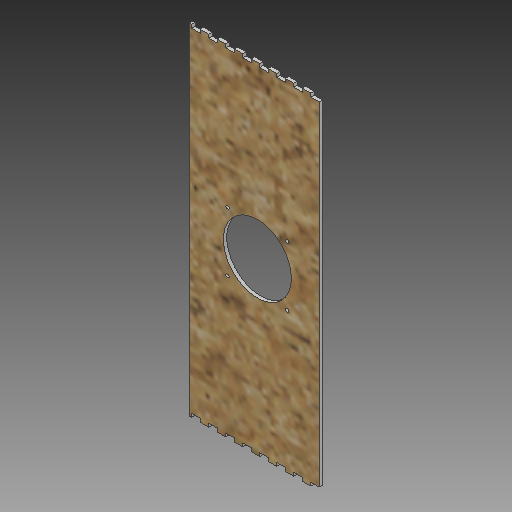
# Autodesk Inventor part: задняя стенка
Saved by Autodesk Inventor 2019 (Build 230136000, 136)
## iProperties
Created: 2022-06-28
Part Number: задняя стенка
Material: Типовые
Document SubType Name: Modeling
Designer: korsh
Density: 1 g/cm^3
Appearance: По умолчанию
Author: korsh
Autodesk Inventor part; units mm, degrees
ref_plane "YZ Plane" through (0, 0, 0) normal (1, 0, 0) x (0, 1, 0)
ref_plane "XZ Plane" through (0, 0, 0) normal (0, 1, 0) x (-1, 0, 0)
ref_plane "XY Plane" through (0, 0, 0) normal (0, 0, 1) x (1, 0, 0)
sketch "Эскиз1" plane through (0, 0, 0) normal (0, 0, 1) x (1, 0, 0)
  circle A0 centre (0, 0) radius 40 projected
  circle A1 centre (35, 35) radius 2 projected
  circle A2 centre (-35, 35) radius 2 projected
  circle A3 centre (-35, -35) radius 2 projected
  circle A4 centre (35, -35) radius 2 projected
  line L0 (72.777, 200) -> (-80, 200)
  line L1 (-80, 200) -> (-80, -200)
  line L2 (-80, -200) -> (72.777, -200)
  line L3 (72.777, -200) -> (72.777, 200)
  point P0 (0, 0)
  dimension "d0" = 400
  dimension "d1" = 200
  dimension "d2" = 80
  constraints: 8 end point, 2 parallel, 1 horizontal, 1 perpendicular
  measures "d0" distance of L2.end L0.start
  measures "d1" distance from line of point (0, 0) L2
  measures "d2" distance from line of L1 point (0, 0)
extrude "Выдавливание1" add sketch "Эскиз1" along normal blind 4
sketch "Эскиз3" plane through (0, 0, 4) normal (0, 0, 1) x (1, 0, 0)
  line L0 (72.777, 200) -> (62.777, 200)
  line L1 (62.777, 200) -> (62.777, 196)
  line L2 (62.777, 196) -> (72.777, 196)
  line L3 (72.777, 196) -> (72.777, 200)
  line L4 (72.777, 200) -> (-80, 200) projected
  line L5 (52.777, 200) -> (42.777, 200)
  line L6 (42.777, 200) -> (42.777, 196)
  line L7 (42.777, 196) -> (52.777, 196)
  line L8 (52.777, 196) -> (52.777, 200)
  line L9 (32.777, 200) -> (22.777, 200)
  line L10 (22.777, 200) -> (22.777, 196)
  line L11 (22.777, 196) -> (32.777, 196)
  line L12 (32.777, 196) -> (32.777, 200)
  line L13 (12.777, 200) -> (2.777, 200)
  line L14 (2.777, 200) -> (2.777, 196)
  line L15 (2.777, 196) -> (12.777, 196)
  line L16 (12.777, 196) -> (12.777, 200)
  line L17 (-7.223, 200) -> (-17.223, 200)
  line L18 (-17.223, 200) -> (-17.223, 196)
  line L19 (-17.223, 196) -> (-7.223, 196)
  line L20 (-7.223, 196) -> (-7.223, 200)
  line L21 (-27.223, 200) -> (-37.223, 200)
  line L22 (-37.223, 200) -> (-37.223, 196)
  line L23 (-37.223, 196) -> (-27.223, 196)
  line L24 (-27.223, 196) -> (-27.223, 200)
  line L25 (-47.223, 200) -> (-57.223, 200)
  line L26 (-57.223, 200) -> (-57.223, 196)
  line L27 (-57.223, 196) -> (-47.223, 196)
  line L28 (-47.223, 196) -> (-47.223, 200)
  line L29 (-67.223, 200) -> (-77.223, 200)
  line L30 (-77.223, 200) -> (-77.223, 196)
  line L31 (-77.223, 196) -> (-67.223, 196)
  line L32 (-67.223, 196) -> (-67.223, 200)
  line L33 (0, 0) -> (123.2904, 0) construction
  line L34 (72.777, -200) -> (62.777, -200)
  line L35 (62.777, -200) -> (62.777, -196)
  line L36 (62.777, -196) -> (72.777, -196)
  line L37 (72.777, -196) -> (72.777, -200)
  line L38 (72.777, -200) -> (-80, -200)
  line L39 (52.777, -200) -> (42.777, -200)
  line L40 (42.777, -200) -> (42.777, -196)
  line L41 (42.777, -196) -> (52.777, -196)
  line L42 (52.777, -196) -> (52.777, -200)
  line L43 (32.777, -200) -> (22.777, -200)
  line L44 (22.777, -200) -> (22.777, -196)
  line L45 (22.777, -196) -> (32.777, -196)
  line L46 (32.777, -196) -> (32.777, -200)
  line L47 (12.777, -200) -> (2.777, -200)
  line L48 (2.777, -200) -> (2.777, -196)
  line L49 (2.777, -196) -> (12.777, -196)
  line L50 (12.777, -196) -> (12.777, -200)
  line L51 (-7.223, -200) -> (-17.223, -200)
  line L52 (-17.223, -200) -> (-17.223, -196)
  line L53 (-17.223, -196) -> (-7.223, -196)
  line L54 (-7.223, -196) -> (-7.223, -200)
  line L55 (-27.223, -200) -> (-37.223, -200)
  line L56 (-37.223, -200) -> (-37.223, -196)
  line L57 (-37.223, -196) -> (-27.223, -196)
  line L58 (-27.223, -196) -> (-27.223, -200)
  line L59 (-47.223, -200) -> (-57.223, -200)
  line L60 (-57.223, -200) -> (-57.223, -196)
  line L61 (-57.223, -196) -> (-47.223, -196)
  line L62 (-47.223, -196) -> (-47.223, -200)
  line L63 (-67.223, -200) -> (-77.223, -200)
  line L64 (-77.223, -200) -> (-77.223, -196)
  line L65 (-77.223, -196) -> (-67.223, -196)
  line L66 (-67.223, -196) -> (-67.223, -200)
  point P0 (-87.223, 200)
  point P1 (-87.223, -200)
  dimension "d7" = 10
  dimension "d8" = 4
  dimension "d11" = 20
  constraints: 132 end point, 34 symmetric about line, 3 horizontal, 2 parallel, 1 perpendicular, 56 other
  measures "d7" distance of L2.end L1.end
  measures "d8" distance of L1.end L0.end
  measures "d11" distance of L1.end L6.end
extrude "Выдавливание2" cut sketch "Эскиз3" against normal blind 4
equation "\"d1\" = 0.5 * d0"
